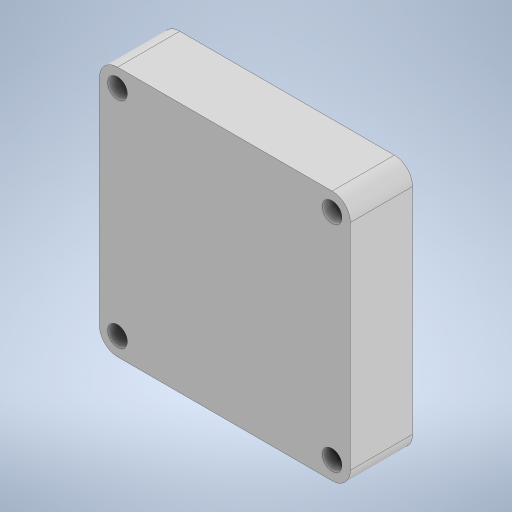
# Autodesk Inventor part: GehauseGenerator_GehauseVorlage
Saved by Autodesk Inventor 2023 (Build 270158000, 158)
## iProperties
Created: 2023-12-25
Part Number: GehauseGenerator_GehauseVorlage
Material: Generisch
Document SubType Name: Modeling
Designer: nfp
Density: 1 g/cm^3
Appearance: Vorgabe
Author: nfp
Autodesk Inventor part; units mm, degrees
ref_plane "YZ Plane" through (0, 0, 0) normal (1, 0, 0) x (0, 1, 0)
ref_plane "XZ Plane" through (0, 0, 0) normal (0, 1, 0) x (-1, 0, 0)
ref_plane "XY Plane" through (0, 0, 0) normal (0, 0, 1) x (1, 0, 0)
sketch "Skizze1" plane through (0, 0, 0) normal (0, 0, 1) x (1, 0, 0)
  line L0 (45, 50) -> (-45, 50)
  line L1 (-50, 45) -> (-50, -45)
  line L2 (-45, -50) -> (45, -50)
  line L3 (50, -45) -> (50, 45)
  line L4 (50, 50) -> (-50, -50) construction
  line L5 (-50, 50) -> (50, -50) construction
  arc A0 (45, -50) -> (50, -45) centre (45, -45) ccw
  arc A1 (-50, -45) -> (-45, -50) centre (-45, -45) ccw
  arc A2 (-45, 50) -> (-50, 45) centre (-45, 45) ccw
  arc A3 (50, 45) -> (45, 50) centre (45, 45) ccw
  line L6 (45, -50.6) -> (-45, -50.6)
  arc A4 (-50.6, -45) -> (-45, -50.6) centre (-45, -45) ccw
  line L7 (-50.6, -45) -> (-50.6, 45)
  arc A5 (-45, 50.6) -> (-50.6, 45) centre (-45, 45) ccw
  line L8 (-45, 50.6) -> (45, 50.6)
  arc A6 (50.6, 45) -> (45, 50.6) centre (45, 45) ccw
  line L9 (50.6, 45) -> (50.6, -45)
  arc A7 (45, -50.6) -> (50.6, -45) centre (45, -45) ccw
  line L10 (-45, -52.6) -> (45, -52.6)
  arc A8 (45, -52.6) -> (52.6, -45) centre (45, -45) ccw
  line L11 (52.6, -45) -> (52.6, 45)
  arc A9 (52.6, 45) -> (45, 52.6) centre (45, 45) ccw
  line L12 (45, 52.6) -> (-45, 52.6)
  arc A10 (-45, 52.6) -> (-52.6, 45) centre (-45, 45) ccw
  line L13 (-52.6, 45) -> (-52.6, -45)
  arc A11 (-52.6, -45) -> (-45, -52.6) centre (-45, -45) ccw
  point P0 (0, 0)
  point P1 (0, 0)
  dimension "d0" = 100
  dimension "d1" = 100
  dimension "d2" = 5
  dimension "d3" = 0.6
  dimension "d4" = 2
  constraints: 28 end point, 24 point on circle, 12 centre point, 8 point on line, 8 tangent, 6 parallel, 3 equal radius, 3 perpendicular, 2 midpoint, 1 coincident, 1 horizontal, 14 other
  measures "d0" distance of L4.end L5.end
  measures "d1" distance of L5.end L4.start
  measures "d2" radius of A0
  measures "d3" distance between parallel lines of L2 L6
  measures "d4" distance between parallel lines of L6 L10
extrude "Extrusion1" add sketch "Skizze1" against normal blind 0.5 contours A11 L13 A10 L12 A9 L11 A8 L10
sketch "Skizze2" plane through (0, 0, 0) normal (0, 0, 1) x (1, 0, 0)
  line L0 (45, 52.6) -> (-45, 52.6) projected
  arc A0 (52.6, 45) -> (45, 52.6) centre (45, 45) ccw projected
  line L1 (52.6, -45) -> (52.6, 45) projected
  arc A1 (45, -52.6) -> (52.6, -45) centre (45, -45) ccw projected
  line L2 (-45, -52.6) -> (45, -52.6) projected
  arc A2 (-52.6, -45) -> (-45, -52.6) centre (-45, -45) ccw projected
  line L3 (-52.6, 45) -> (-52.6, -45) projected
  arc A3 (-45, 52.6) -> (-52.6, 45) centre (-45, 45) ccw projected
  line L4 (-41.4504, 47.6) -> (0, 47.6)
  line L5 (-47.6, 0) -> (-47.6, 41.4504)
  circle A4 centre (-45, 45) radius 1.7
  line L6 (-45, 50.6) -> (45, 50.6) projected
  line L7 (-50.6, -45) -> (-50.6, 45) projected
  arc A5 (-47.6, 41.4504) -> (-41.4504, 47.6) centre (-45, 45) ccw
  line L8 (-45, 52.6) -> (45, 52.6) construction
  line L9 (0, 52.6) -> (0, -52.6) construction
  line L10 (45, -52.6) -> (-45, -52.6) construction
  line L11 (-52.6, 0) -> (52.6, 0) construction
  line L12 (41.4504, 47.6) -> (0, 47.6)
  line L13 (47.6, 0) -> (47.6, 41.4504)
  circle A6 centre (45, 45) radius 1.7
  arc A7 (41.4504, 47.6) -> (47.6, 41.4504) centre (45, 45) ccw
  line L14 (-41.4504, -47.6) -> (0, -47.6)
  line L15 (-47.6, 0) -> (-47.6, -41.4504)
  circle A8 centre (-45, -45) radius 1.7
  arc A9 (-41.4504, -47.6) -> (-47.6, -41.4504) centre (-45, -45) ccw
  line L16 (47.6, 0) -> (47.6, -41.4504)
  arc A10 (47.6, -41.4504) -> (41.4504, -47.6) centre (45, -45) ccw
  circle A11 centre (45, -45) radius 1.7
  line L17 (41.4504, -47.6) -> (0, -47.6)
  point P0 (0, 0)
  dimension "d11" = 5
  dimension "d13" = 5
  dimension "d15" = 3.4
  dimension "d16" = 5.6
  dimension "d17" = 5.6
  dimension "d18" = 4.4
  constraints: 20 end point, 14 symmetric about line, 8 centre point, 8 point on circle, 4 coincident, 4 midpoint, 2 point on line, 1 horizontal, 6 other
  measures "d11" distance between parallel lines of L0 L4
  measures "d13" distance between parallel lines of L3 L5
  measures "d15" diameter of A4
  measures "d16" distance from line of L6 A4.centre
  measures "d17" distance from line of L7 A4.centre
  measures "d18" radius of A5
extrude "Extrusion2" add sketch "Skizze2" along normal blind 20.6
sketch "Skizze3" plane through (0, 0, 20.6) normal (0, 0, 1) x (1, 0, 0)
  line L0 (-52.6, 45) -> (-52.6, -45) projected
  arc A0 (-52.6, -45) -> (-45, -52.6) centre (-45, -45) ccw projected
  line L1 (-45, -52.6) -> (45, -52.6) projected
  arc A1 (45, -52.6) -> (52.6, -45) centre (45, -45) ccw projected
  line L2 (52.6, -45) -> (52.6, 45) projected
  arc A2 (52.6, 45) -> (45, 52.6) centre (45, 45) ccw projected
  line L3 (45, 52.6) -> (-45, 52.6) projected
  arc A3 (-45, 52.6) -> (-52.6, 45) centre (-45, 45) ccw projected
  point P0 (0, 0)
extrude "Extrusion3" add sketch "Skizze3" along normal blind 5
fillet "Rundung1" radius 5 8 edges at (-47.6, 41.4504, 10.3) (-41.4504, 47.6, 10.3) (47.6, 41.4504, 10.3) (41.4504, 47.6, 10.3) (41.4504, -47.6, 10.3) (47.6, -41.4504, 10.3) (-41.4504, -47.6, 10.3) (-47.6, -41.4504, 10.3)
fillet "Rundung2" radius 5 16 edges at (-46.5612, 38.9625, 20.6) (-41.8887, 41.8887, 20.6) (-38.9625, 46.5612, 20.6) (0, 47.6, 20.6) (38.9625, 46.5612, 20.6) (41.8887, 41.8887, 20.6) (46.5612, 38.9625, 20.6) (47.6, 0, 20.6) (46.5612, -38.9625, 20.6) (41.8887, -41.8887, 20.6) (38.9625, -46.5612, 20.6) (0, -47.6, 20.6) (-38.9625, -46.5612, 20.6) (-41.8887, -41.8887, 20.6) (-46.5612, -38.9625, 20.6) (-47.6, 0, 20.6)
sketch "Skizze4" plane through (0, 0, 25.6) normal (0, 0, 1) x (1, 0, 0)
  arc A0 (-45, 52.6) -> (-52.6, 45) centre (-45, 45) ccw projected
  arc A1 (52.6, 45) -> (45, 52.6) centre (45, 45) ccw projected
  arc A2 (45, -52.6) -> (52.6, -45) centre (45, -45) ccw projected
  arc A3 (-52.6, -45) -> (-45, -52.6) centre (-45, -45) ccw projected
  circle A4 centre (-45, 45) radius 1.7 projected
  circle A5 centre (-45, 45) radius 4.1
  circle A6 centre (45, 45) radius 4.1
  circle A7 centre (45, -45) radius 1.7 projected
  circle A8 centre (45, -45) radius 4.1
  circle A9 centre (-45, -45) radius 1.7 projected
  circle A10 centre (-45, -45) radius 4.1
  point P0 (0, 0)
  dimension "d25" = 8.2
  dimension "d26" = 8.2
  dimension "d27" = 8.2
  dimension "d28" = 8.2
  constraints: 4 centre point, 4 coincident
  measures "d25" diameter of A5
  measures "d26" diameter of A10
  measures "d27" diameter of A6
  measures "d28" diameter of A8
extrude "ExtrusionSchraubenKopf" cut sketch "Skizze4" against normal blind 7.6 contours A4 | A5 | A6 | A7 | A8 | A9 | A10
sketch "Skizze5" plane through (0, 0, 0) normal (0, 0, -1) x (-1, 0, 0)
  circle A0 centre (45, 45) radius 1.7 projected
  circle A1 centre (45, -45) radius 1.7 projected
  circle A2 centre (-45, -45) radius 1.7 projected
  circle A3 centre (-45, 45) radius 1.7 projected
  point P0 (0, 0)
extrude "ExtrusionSchraubenLoch" cut sketch "Skizze5" against normal up to surface (25.6 mm away)
equation "\"d0\" = BP"
equation "\"d1\" = LP"
equation "\"d2\" = REP"
equation "\"d3\" = TM"
equation "\"d9\" = -0.5 * TM + 0.5 * HPt"
equation "\"d11\" = DW"
equation "\"d13\" = DW"
equation "\"d15\" = DL"
equation "\"d16\" = REP + TM"
equation "\"d17\" = REP + TM"
equation "\"d19\" = HPb + TM"
equation "\"d21\" = DW"
equation "\"d23\" = RR"
equation "\"d24\" = RR"
equation "\"d25\" = SKD + 2 * TM"
equation "\"d26\" = SKD + 2 * TM"
equation "\"d27\" = SKD + 2 * TM"
equation "\"d28\" = SKD + 2 * TM"
equation "\"d29\" = SKH + TM"
equation "\"BP\" = 100"
equation "\"LP\" = 100"
equation "\"REP\" = 5"
equation "\"TM\" = 0.6"
equation "\"DW\" = 5"
equation "\"DL\" = 3.4"
equation "\"HPt\" = 1.6"
equation "\"HPb\" = 20"
equation "\"RR\" = 5"
equation "\"SKD\" = 7"
equation "\"SKH\" = 7"
